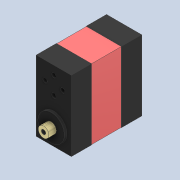
# Autodesk Inventor part: サーボモーター25kgcmサーボモータ
Saved by Autodesk Inventor 2021.2 (Build 252289000, 289)
## iProperties
Created: 2020-02-02
Part Number: サーボモーター25kgcmサーボモータ
Material: アルミニウム 6061
Document SubType Name: Modeling
Designer: yuta2
Density: 2.02338 g/cm^3
Appearance: ゴム - 黒
Mass: 65 g
Surface Area: 71.4194 cm^2
Volume: 32.1244 cm^3
Author: yuta2
Autodesk Inventor part; units mm, degrees
ref_plane "YZ Plane" through (0, 0, 0) normal (1, 0, 0) x (0, 1, 0)
ref_plane "XZ Plane" through (0, 0, 0) normal (0, 1, 0) x (-1, 0, 0)
ref_plane "XY Plane" through (0, 0, 0) normal (0, 0, 1) x (1, 0, 0)
sketch "スケッチ1" plane through (0, 0, 0) normal (1, 0, 0) x (0, 1, 0)
  line L0 (0, 0) -> (40, 0)
  line L1 (40, 0) -> (40, -40)
  line L2 (40, -40) -> (0, -40)
  line L3 (0, -40) -> (0, 0)
  dimension "d0" = 40
  dimension "d1" = 40
  constraints: 8 end point, 2 parallel, 1 horizontal, 1 perpendicular
  measures "d0" distance of L1.end L2.end
  measures "d1" distance of L0.end L1.end
extrude "押し出し1" add sketch "スケッチ1" along normal blind 20
sketch "スケッチ2" plane through (0, 0, 0) normal (0, 0, 1) x (1, 0, 0)
  circle A0 centre (10, 10) radius 7.5
  line L0 (0, 0) -> (20, 0) projected
  line L1 (0, 40) -> (0, 0) projected
  dimension "d4" = 15
  dimension "d5" = 10
  dimension "d6" = 10
  constraints: 1 centre point
  measures "d4" diameter of A0
  measures "d5" distance from line of L0 A0.centre
  measures "d6" distance from line of L1 A0.centre
extrude "押し出し2" add sketch "スケッチ2" along normal blind 1.5
sketch "スケッチ3" plane through (0, 0, -40) normal (0, 0, -1) x (-1, 0, 0)
  circle A0 centre (-10, 10) radius 7.5
  line L0 (0, 0) -> (-20, 0) projected
  line L1 (0, 0) -> (0, 40) projected
  dimension "d9" = 15
  dimension "d10" = 10
  dimension "d11" = 10
  constraints: 1 centre point
  measures "d9" diameter of A0
  measures "d10" distance from line of L0 A0.centre
  measures "d11" distance from line of L1 A0.centre
extrude "押し出し3" add sketch "スケッチ3" along normal blind 1.5
sketch "スケッチ4" plane through (20, 0, 0) normal (1, 0, 0) x (0, 0, -1)
  line L0 (40, 40) -> (0, 40) projected
  line L1 (20, 40) -> (20, 0)
  line L2 (0, 0) -> (40, 0) projected
  line L3 (11.5, 40) -> (28.5, 40)
  line L4 (28.5, 40) -> (28.5, 0)
  line L5 (28.5, 0) -> (11.5, 0)
  line L6 (11.5, 0) -> (11.5, 40)
  dimension "d14" = 17
  constraints: 10 end point, 2 midpoint, 2 parallel, 2 point on line, 1 horizontal, 1 perpendicular, 1 other
  measures "d14" distance between parallel lines of L4 L6
extrude "押し出し4" cut sketch "スケッチ4" against normal blind 0.1
sketch "スケッチ5" plane through (0, 40, 0) normal (0, 1, 0) x (1, 0, 0)
  line L0 (0, 0) -> (0, 40) projected
  line L1 (0, 20) -> (19.9, 20)
  line L2 (19.9, 11.5) -> (19.9, 28.5) projected
  line L3 (19.9, 11.5) -> (0, 11.5)
  line L4 (0, 11.5) -> (0, 28.5)
  line L5 (0, 28.5) -> (19.9, 28.5)
  line L6 (19.9, 28.5) -> (19.9, 11.5)
  constraints: 10 end point, 2 midpoint, 2 parallel, 1 horizontal, 1 perpendicular, 1 point on line
extrude "押し出し5" cut sketch "スケッチ5" against normal blind 0.1
sketch "スケッチ6" plane through (0, 0, 0) normal (-1, 0, 0) x (0, 0, 1)
  line L0 (-11.5, 39.9) -> (-28.5, 39.9) projected
  line L1 (-20, 39.9) -> (-20, 0)
  line L2 (-28.5, 0) -> (-11.5, 0) projected
  line L3 (-28.5, 39.9) -> (-11.5, 39.9)
  line L4 (-11.5, 39.9) -> (-11.5, 0)
  line L5 (-11.5, 0) -> (-28.5, 0)
  line L6 (-28.5, 0) -> (-28.5, 39.9)
  point P0 (0, 0)
  constraints: 10 end point, 2 midpoint, 2 parallel, 1 horizontal, 1 perpendicular
extrude "押し出し6" cut sketch "スケッチ6" against normal blind 0.1
sketch "スケッチ7" plane through (0, 0, -40) normal (0, -1, 0) x (1, 0, 0)
  line L0 (0.1, 28.5) -> (0.1, 11.5) projected
  line L1 (20, 28.5) -> (0, 28.5) projected
  line L2 (0.1, 11.5) -> (20, 11.5)
  line L3 (20, 11.5) -> (20, 28.5)
  line L4 (20, 28.5) -> (0.1, 28.5)
  line L5 (0.1, 28.5) -> (0.1, 11.5)
  point P0 (0, 40)
  constraints: 8 end point, 2 parallel, 1 horizontal, 1 perpendicular
extrude "押し出し7" cut sketch "スケッチ7" against normal blind 0.1
sketch "スケッチ8" plane through (0, 0, -40) normal (0, 0, -1) x (-1, 0, 0)
  line L0 (0, 40) -> (-20, 40) projected
  line L1 (-20, 0) -> (-20, 40) projected
  line L2 (0, 0) -> (0, 40) projected
  point P0 (-17.5, 37.5)
  point P1 (-2.5, 37.5)
  point P2 (-2.5, 22.5)
  point P3 (-17.5, 22.5)
  dimension "d23" = 2.5
  dimension "d24" = 2.5
  dimension "d25" = 2.5
  dimension "d26" = 15
  constraints: 2 horizontal alignment, 2 vertical alignment
  measures "d23" distance from line of L0 point (-2.5, 37.5)
  measures "d24" distance from line of L1 point (-17.5, 37.5)
  measures "d25" distance from line of L2 point (-2.5, 37.5)
  measures "d26" distance of point (-17.5, 22.5) point (-17.5, 37.5)
hole "穴1" at (17.5, 37.5, -40) at (2.5, 37.5, -40) at (2.5, 22.5, -40) at (17.5, 22.5, -40) direction (0, 0, 1) diameter 2.5 depth 8 tip angle 118
sketch "スケッチ9" plane through (0, 0, 0) normal (0, 0, 1) x (1, 0, 0)
  line L0 (0, 40) -> (20, 40) projected
  line L1 (20, 40) -> (20, 0) projected
  line L2 (0, 40) -> (0, 0) projected
  circle A0 centre (10, 30) radius 5
  point P0 (10, 25)
  point P1 (5, 30)
  point P2 (15, 30)
  point P3 (10, 35)
  dimension "d48" = 10
  dimension "d49" = 10
  dimension "d50" = 10
  constraints: 4 point on circle, 2 horizontal alignment, 2 vertical alignment, 1 centre point
  measures "d48" diameter of A0
  measures "d49" distance from line of L1 A0.centre
  measures "d50" distance from line of L0 A0.centre
hole "穴2" at (10, 25, 0) at (5, 30, 0) at (15, 30, 0) at (10, 35, 0) direction (0, 0, -1) diameter 2.5 depth 8 tip angle 118
sketch "スケッチ10" plane through (10, 10, 1.5) normal (0, 0, 1) x (1, 0, 0)
  circle A0 centre (0, 0) radius 7.5 projected
  circle A1 centre (0, 0) radius 3
  point P0 (-10, -10)
  dimension "d45" = 6
  constraints: 1 centre point, 1 coincident
  measures "d45" diameter of A1
extrude "押し出し8" add sketch "スケッチ10" along normal blind 4.3 contours A1
sketch "スケッチ11" plane through (10, 10, -41.5) normal (0, 0, -1) x (-1, 0, 0)
  circle A0 centre (0, 0) radius 7.5 projected
  circle A1 centre (0, 0) radius 3
  circle A2 centre (0, 0) radius 1
  point P0 (10, -10)
  dimension "d51" = 6
  dimension "d54" = 2
  constraints: 2 centre point, 2 coincident
  measures "d51" diameter of A1
  measures "d54" diameter of A2
extrude "押し出し9" add sketch "スケッチ11" along normal blind 5.5 contours A1
sketch "スケッチ12" plane through (0, 0, -40) normal (0, -1, 0) x (1, 0, 0)
  line L0 (20, 11.5) -> (0, 11.5) projected
  line L1 (13.25, 11.5) -> (6.75, 11.5)
  line L2 (6.75, 11.5) -> (6.75, 7)
  line L3 (6.75, 7) -> (13.25, 7)
  line L4 (13.25, 7) -> (13.25, 11.5)
  point P0 (0, 40)
  point P1 (6.75, 11.5)
  point P2 (10, 11.5)
  dimension "d55" = 6.5
  dimension "d56" = 4.5
  constraints: 8 end point, 2 midpoint, 2 parallel, 1 horizontal, 1 perpendicular, 1 point on line
  measures "d55" distance of L2.end L3.end
  measures "d56" distance of L1.end L2.end
extrude "押し出し10" add sketch "スケッチ12" along normal blind 5
sketch "スケッチ13" plane through (10, 10, 5.8) normal (0, 0, 1) x (1, 0, 0)
  point P0 (0, 0)
hole "穴3" at (10, 10, 5.8) direction (0, 0, -1) diameter 2.459 depth 8 tip angle 120 thread size "M3x0.5" class "6H" standard "ISO Metric profile"
